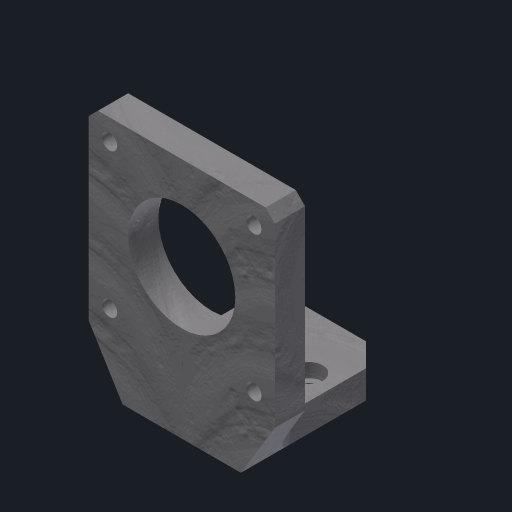
# Autodesk Inventor part: ACOPLE_NEMA_PUERTA
Saved by Autodesk Inventor 2024.3 (Build 283343000, 343)
## iProperties
Created: 2024-06-23
Part Number: ACOPLE_NEMA_PUERTA
Material: Steel, Mild, Welded
Document SubType Name: Modeling
Designer: Niler
Density: 7.85 g/cm^3
Appearance: Weld - Steel Mild
Author: Niler
Autodesk Inventor part; units mm, degrees
ref_plane "YZ Plane" through (0, 0, 0) normal (1, 0, 0) x (0, 1, 0)
ref_plane "XZ Plane" through (0, 0, 0) normal (0, 1, 0) x (-1, 0, 0)
ref_plane "XY Plane" through (0, 0, 0) normal (0, 0, 1) x (1, 0, 0)
sketch "Sketch1" plane through (0, 0, 0) normal (0, 0, 1) x (1, 0, 0)
  line L0 (-20, -20) -> (20, -20)
  line L1 (20, -20) -> (20, 20)
  line L2 (20, 20) -> (-20, 20)
  line L3 (-20, 20) -> (-20, -20)
  line L4 (-20, -20) -> (20, 20) construction
  line L5 (20, -20) -> (-20, 20) construction
  line L6 (-15.5, -15.5) -> (15.5, -15.5) construction
  line L7 (15.5, -15.5) -> (15.5, 15.5) construction
  line L8 (15.5, 15.5) -> (-15.5, 15.5) construction
  line L9 (-15.5, 15.5) -> (-15.5, -15.5) construction
  line L10 (-15.5, -15.5) -> (15.5, 15.5) construction
  line L11 (15.5, -15.5) -> (-15.5, 15.5) construction
  circle A0 centre (-15.5, 15.5) radius 1.65
  circle A1 centre (15.5, 15.5) radius 1.65
  circle A2 centre (15.5, -15.5) radius 1.65
  circle A3 centre (-15.5, -15.5) radius 1.65
  circle A4 centre (0, 0) radius 11.5
  dimension "d0" = 40
  dimension "d1" = 40
  dimension "d2" = 31
  dimension "d3" = 31
  dimension "d4" = 3.3
  dimension "d5" = 23
  constraints: 24 end point, 5 centre point, 5 coincident, 4 midpoint, 4 parallel, 3 equal radius, 2 horizontal, 2 perpendicular
  measures "d0" distance of L2.end L1.end
  measures "d1" distance of L2.end L0.start
  measures "d2" distance of L8.end L7.end
  measures "d3" distance of L7.end L6.end
  measures "d4" diameter of A0
  measures "d5" diameter of A4
extrude "Extrusion1" add sketch "Sketch1" along normal blind 6.5
sketch "Sketch2" plane through (0, 0, 6.5) normal (0, 0, 1) x (1, 0, 0)
  line L0 (-20, -20) -> (20, -20) projected
  line L1 (-20, -20) -> (20, -20) projected
  line L2 (-12.7, -20) -> (12.7, -20)
  line L3 (12.7, -20) -> (12.7, -32)
  line L4 (12.7, -32) -> (-12.7, -32)
  line L5 (-12.7, -32) -> (-12.7, -20)
  line L6 (20, -20) -> (12.7, -32)
  line L7 (-12.7, -32) -> (-20, -20)
  point P0 (0, 0)
  point P1 (0, -32)
  point P2 (0, -20)
  dimension "d8" = 25.4
  dimension "d9" = 12
  constraints: 12 end point, 2 midpoint, 2 parallel, 1 horizontal, 1 perpendicular, 1 point on line, 1 vertical alignment
  measures "d8" distance between parallel lines of L3 L5
  measures "d9" distance of L2.end L3.end
extrude "Extrusion2" add sketch "Sketch2" against normal up to surface (6.5 mm away)
sketch "Sketch3" plane through (0, 0, 0) normal (0, 0, -1) x (-1, 0, 0)
  line L0 (-20, -20) -> (-20, 20) projected
  line L1 (-20, -20) -> (-12.7, -32) projected
  line L2 (-12.7, -32) -> (12.7, -32) projected
  line L3 (12.7, -32) -> (20, -20) projected
  line L4 (20, 20) -> (20, -20) projected
  line L5 (-20, 20) -> (20, 20) projected
  circle A0 centre (15.5, 15.5) radius 1.65 projected
  circle A1 centre (-15.5, 15.5) radius 1.65 projected
  circle A2 centre (-15.5, -15.5) radius 1.65 projected
  circle A3 centre (15.5, -15.5) radius 1.65 projected
  circle A4 centre (0, 0) radius 11.5 projected
  line L6 (-12.7, -32) -> (12.7, -32)
  line L7 (12.7, -32) -> (12.7, -26)
  line L8 (12.7, -26) -> (-12.7, -26)
  line L9 (-12.7, -26) -> (-12.7, -32)
  dimension "d12" = 6
  constraints: 8 end point, 2 parallel, 1 horizontal, 1 perpendicular
  measures "d12" distance between parallel lines of L2 L8
extrude "Extrusion3" add sketch "Sketch3" along normal blind 25.4 contours L9 L8 L7 L2
fillet "Fillet1" radius 2 1 edges at (0, -26, 0)
fillet "Fillet2" radius 4 4 edges at (12.7, -25, 0) (12.7, -29, 0) (-12.7, -25, 0) (-12.7, -29, 0)
chamfer "Chamfer1" distance 2 angle 45 2 edges at (20, 20, 3.25) (-20, 20, 3.25)
chamfer "Chamfer2" distance 5 angle 45 2 edges at (12.7, -29, -25.4) (-12.7, -29, -25.4)
sketch "Sketch4" plane through (-13.2359, -26, -2) normal (0, 1, 0) x (1, 0, 0)
  line L0 (0.5359, 18.4) -> (5.5359, 23.4) projected
  line L1 (0.5359, 2) -> (0.5359, 18.4) projected
  line L2 (26.4718, 0) -> (0, 0) projected
  line L3 (25.9359, 2) -> (25.9359, 18.4) projected
  line L4 (20.9359, 23.4) -> (25.9359, 18.4) projected
  line L5 (5.5359, 23.4) -> (20.9359, 23.4) projected
  circle A0 centre (5.7359, 11.4) radius 1.65
  circle A1 centre (20.7359, 11.4) radius 1.65
  arc A2 (0, 0) -> (0.5359, 2) centre (-3.4641, 2) ccw projected
  arc A3 (25.9359, 2) -> (26.4718, 0) centre (29.9359, 2) ccw projected
  line L6 (5.7359, 11.4) -> (20.7359, 11.4) construction
  line L7 (5.5359, 23.4) -> (20.9359, 23.4) construction
  point P0 (13.2359, -2)
  point P1 (13.2359, 23.4)
  point P2 (13.2359, 11.4)
  point P3 (13.2359, 23.4)
  dimension "d23" = 3.3
  dimension "d24" = 15
  dimension "d25" = 12
  constraints: 3 midpoint, 2 centre point, 2 end point, 1 equal radius, 1 horizontal, 1 horizontal alignment, 1 vertical alignment
  measures "d23" diameter of A0
  measures "d24" distance of L6.start L6.end
  measures "d25" distance from line of L5 L6.end
extrude "Extrusion4" cut sketch "Sketch4" against normal through all contours A0 | A1
sketch "Sketch5" plane through (-13.2359, -26, -2) normal (0, 1, 0) x (1, 0, 0)
  circle A0 centre (20.7359, 11.4) radius 1.65 projected
  circle A1 centre (20.7359, 11.4) radius 2.9
  circle A2 centre (5.7359, 11.4) radius 1.65 projected
  circle A3 centre (5.7359, 11.4) radius 2.9
  point P0 (13.2359, -2)
  point P1 (13.2359, 13)
  dimension "d31" = 5.8
  constraints: 2 centre point, 2 coincident, 1 equal radius
  measures "d31" diameter of A3
extrude "Extrusion5" cut sketch "Sketch5" against normal blind 3 contours A0 | A1 | A2 | A3
body "Solid1"
